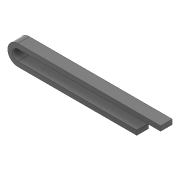
# Autodesk Inventor part: J15BF.1.40_Xaxis
Saved by Autodesk Inventor 2020 (Build 240168000, 168)
## iProperties
Created: 2020-06-16
Part Number: J15BF.1.40_Xaxis
Material: Generic
Document SubType Name: Modeling
Designer: hirohouse
Density: 1 g/cm^3
Appearance: Default
Author: hirohouse
Autodesk Inventor part; units mm, degrees
ref_plane "YZ Plane" through (0, 0, 0) normal (1, 0, 0) x (0, 1, 0)
ref_plane "XZ Plane" through (0, 0, 0) normal (0, 1, 0) x (-1, 0, 0)
ref_plane "XY Plane" through (0, 0, 0) normal (0, 0, 1) x (1, 0, 0)
sketch "Sketch1" plane through (0, 0, 0) normal (0, 0, 1) x (1, 0, 0)
  circle A0 centre (0, 0) radius 42.5
  line L0 (0, -42.5) -> (500, -42.5)
  line L1 (500, -42.5) -> (500, -22.5)
  line L2 (500, -22.5) -> (0, -22.5)
  line L3 (0, -22.5) -> (0, -42.5)
  line L4 (0, 42.5) -> (600, 42.5)
  line L5 (600, 42.5) -> (600, 22.5)
  line L6 (600, 22.5) -> (0, 22.5)
  line L7 (0, 22.5) -> (0, 42.5)
  circle A1 centre (0, 0) radius 22.5
  point P0 (0, -22.5)
  point P1 (0, 22.5)
  dimension "d0" = 85
  dimension "d1" = 20
  dimension "d2" = 20
  dimension "d4" = 500
  dimension "d9" = 600
  constraints: 16 end point, 4 parallel, 2 centre point, 2 coincident, 2 horizontal, 2 perpendicular, 2 point on circle, 1 point on line, 1 tangent
  measures "d0" diameter of A0
  measures "d1" distance of L4.end L5.end
  measures "d2" distance of L0.end L1.end
  measures "d4" distance from line of L1 point (0, 0)
  measures "d9" distance of L4.start L4.end
extrude "Extrusion1" add sketch "Sketch1" along normal blind 49 contours L7 A1 L3 A0 | L4 L5 L6 A0 | A0 L6 L7 | L3 L2 A0 | A0 L2 L1 L0
body "Solid1"
